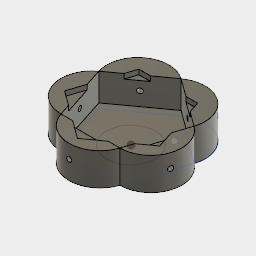
胸花 (Autodesk Fusion 360 design; units mm, degrees)
Autodesk Fusion 360 part; units mm, degrees
sketch "草图1" plane through (0, 0, 0) normal (0, 1, 0) x (1, 0, 0)
  circle A0 centre (0, 0) radius 15
  line L0 (18.1586, -25.0036) -> (29.3912, 9.5433)
  line L1 (29.3912, 9.5433) -> (0.0061, 30.9017)
  line L2 (0.0061, 30.9017) -> (-29.3874, 9.555)
  line L3 (-29.3874, 9.555) -> (-18.1685, -24.9964)
  line L4 (-18.1685, -24.9964) -> (18.1586, -25.0036)
  arc A1 (29.3912, 9.5433) -> (0.0061, 30.9017) centre (11.2288, 15.4486) ccw
  dimension "d1" = 30
  dimension "d2" = 25
  measures "d1" diameter of A0
  measures "d2" distance of A0.centre L4
extrude "拉伸1" add sketch "草图1" along normal blind 20 contours L1 A1 makes body 1
pattern_circular "C-阵列1" count 5 over 360 about axis through (0, 0, 0) along (0, 1, 0) of bodies 1 makes body 2 at (-14.2646, 13.3333, -34.3076) makes body 3 at (-31.7135, 13.3333, 19.3583) makes body 4 at (-17.8559, 6.6667, 25.884) makes body 5 at (19.0994, 6.6667, 24.9806)
extrude "拉伸2" add sketch "草图1" along normal blind 3 contours A0 | L0 L1 L2 L3 L4 bodies 1 2 3 4 5
cylinder "圆柱体基本要素1" add diameter 3 height 60 placed x (1, 0, 0) y (0, 1, 0) z (0, 0, 1) at (90, 0, 0) separate body makes body 6
move_body "对齐1" bodies 6 to x (-1, 0, -0.000199) y (0, -1, 0) z (-0.000199, 0, 1) at (90.007, 11.5, -34.9821)
move_body "移动1" bodies 6 to x (1, 0, 0) y (0, 1, 0) z (0, 0, 1) at (0, 0, 40)
pattern_circular "C-阵列2" count 5 over 360 about axis through (0, 0, 0) along (0, 1, 0) of bodies 6 makes body 7 at (42.3357, 11.6494, 15.3261) makes body 8 at (14.8431, 10.0116, -20.1175) makes body 9 at (-15.4055, 10.2821, -19.7091) makes body 10 at (-23.5242, 12.76, 8.5023)
combine "合并1" operation cut target body 1 tool bodies 6 8 10 9 7
sketch "草图3" plane through (0, 0, 0) normal (0, 1, 0) x (1, 0, 0)
  line L0 (69.9416, -30.9016) -> (99.3712, -9.6047)
  line L1 (99.3712, -9.6047) -> (88.2108, 24.9656)
  line L2 (88.2108, 24.9656) -> (51.8837, 25.0343)
  line L3 (51.8837, 25.0343) -> (40.5927, -9.4936)
  line L4 (40.5927, -9.4936) -> (69.9416, -30.9016)
  point P0 (70, 0)
  dimension "d13" = 25
  measures "d13" distance of P0 L4
extrude "拉伸3" add sketch "草图3" along normal blind 3 separate body makes body 11
move_body "对齐2" bodies 11 to x (1, 0, 0) y (0, 1, 0) z (0, 0, 1) at (-69.9819, -3, -2.9337)
move_body "移动2" bodies 11 to x (1, 0, 0) y (0, 1, 0) z (0, 0, 1) at (0, 20, 0)
move_body "移动3" bodies 11 to x (1, 0, 0) y (0, 1, 0) z (0, 0, 1) at (0, 0, 5)
combine "合并2" operation cut target body 1 tool bodies 11
